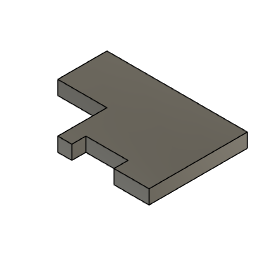
Keychain (Autodesk Fusion 360 design; units mm, degrees)
Autodesk Fusion 360 part; units mm, degrees
sketch "keychain base" plane through (0, 0, 0) normal (0, 0, 1) x (1, 0, 0)
  line L0 (-15, 0) -> (85, 0)
  line L1 (85, 0) -> (85, -70)
  line L2 (85, -70) -> (60, -70)
  line L3 (60, -70) -> (60, -60)
  line L4 (60, -60) -> (50, -60)
  line L5 (50, -60) -> (30, -60)
  line L6 (30, -60) -> (30, -70)
  line L7 (30, -70) -> (20, -70)
  line L8 (20, -70) -> (20, -35)
  line L9 (20, -35) -> (0, -35)
  line L10 (0, -35) -> (-15, -35)
  line L11 (-15, -35) -> (-15, 0)
  constraint horizontal L0
  constraint perpendicular L0 L1
  constraint perpendicular L1 L2
  constraint perpendicular L2 L3
  constraint perpendicular L1 L4
  constraint perpendicular L1 L5
  constraint perpendicular L5 L6
  constraint perpendicular L6 L7
  constraint perpendicular L5 L8
  constraint perpendicular L6 L9
  constraint parallel L0 L10
  constraint perpendicular L0 L11
extrude "Extrude1" add sketch "keychain base" along normal blind 10
named bodies: "keychain"
